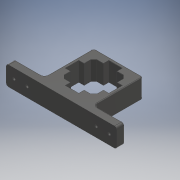
# Autodesk Inventor part: Support moteur
Saved by Autodesk Inventor 2017 (Build 210142000, 142)
## iProperties
Company: FABLAB Frenchmakers
Part Number: Support moteur
Material: Plastique ABS
Document SubType Name: Modeling
Designer: FABLAB Frenchmakers
Density: 1.06 g/cm^3
Appearance: Lisse - Blanc(3)
Mass: 88.0061 g
Surface Area: 230.451 cm^2
Volume: 83.0246 cm^3
Project: 1420 Vauban 3D XL
Catalog Web Link: http://frenchmakers.com/
Stock Number: 1420-05-01
Autodesk Inventor part; units mm, degrees
ref_plane "YZ Plane" through (0, 0, 0) normal (1, 0, 0) x (0, 1, 0)
ref_plane "XZ Plane" through (0, 0, 0) normal (0, 1, 0) x (-1, 0, 0)
sketch "Esquisse1" plane through (0, 0, 0) normal (0, 0, 1) x (1, 0, 0)
  line L0 (-17.3, -21.3) -> (17.3, -21.3)
  line L1 (21.3, -17.3) -> (21.3, 17.3)
  line L2 (17.3, 21.3) -> (-17.3, 21.3)
  line L3 (-21.3, 17.3) -> (-21.3, -17.3)
  line L4 (-21.3, -21.3) -> (21.3, 21.3) construction
  line L5 (21.3, -21.3) -> (-21.3, 21.3) construction
  line L6 (-21.3, 17.3) -> (-17.3, 21.3)
  line L7 (21.3, 17.3) -> (17.3, 21.3)
  line L8 (21.3, -17.3) -> (17.3, -21.3)
  line L9 (-17.3, -21.3) -> (-21.3, -17.3)
  line L10 (-32.3, -32.3) -> (32.3, -32.3)
  line L11 (32.3, -32.3) -> (32.3, 32.3)
  line L12 (32.3, 32.3) -> (-32.3, 32.3)
  line L13 (-32.3, 32.3) -> (-32.3, -32.3)
  line L14 (-32.3, -32.3) -> (32.3, 32.3) construction
  line L15 (32.3, -32.3) -> (-32.3, 32.3) construction
  point P0 (0, 0)
  dimension "d0" = 42.6
  dimension "d1" = 42.6
  dimension "d7" = 4
  dimension "d8" = 4
  dimension "d9" = 4
  dimension "d10" = 4
  dimension "d11" = 4
  dimension "d12" = 4
  dimension "d13" = 4
  dimension "d14" = 4
  dimension "d15" = 11
  dimension "d16" = 11
  constraints: 32 end point, 8 point on line, 4 midpoint, 4 parallel, 2 horizontal, 2 perpendicular
  measures "d0" distance of L5.end L4.end
  measures "d1" distance of L4.end L5.start
  measures "d7" distance of L3.start L5.end
  measures "d8" distance of L2.end L5.end
  measures "d9" distance of L1.end L4.end
  measures "d10" distance of L2.start L4.end
  measures "d11" distance of L1.start L5.start
  measures "d12" distance of L0.end L5.start
  measures "d13" distance of L0.start L4.start
  measures "d14" distance of L3.end L4.start
  measures "d15" distance between parallel lines of L2 L12
  measures "d16" distance between parallel lines of L3 L13
extrude "Extrusion1" add sketch "Esquisse1" along normal mid plane 25
sketch "Esquisse2" plane through (-32.3, -32.3, 12.5) normal (0, -1, 0) x (1, 0, 0)
  line L0 (-40, 0) -> (104.6, 0)
  line L1 (104.6, 0) -> (104.6, -25)
  line L2 (104.6, -25) -> (-40, -25)
  line L3 (-40, -25) -> (-40, 0)
  line L4 (-40, 0) -> (104.6, -25) construction
  line L5 (104.6, 0) -> (-40, -25) construction
  line L6 (0, 0) -> (64.6, 0) projected
  line L7 (64.6, -25) -> (64.6, 0) projected
  point P0 (32.3, -12.5)
  dimension "d17" = 40
  constraints: 12 end point, 2 midpoint, 2 parallel, 1 collinear, 1 horizontal, 1 perpendicular
  measures "d17" distance between parallel lines of L7 L1
extrude "Extrusion2" add sketch "Esquisse2" along normal blind 10
sketch "Esquisse3" plane through (-32.3, -32.3, 12.5) normal (0, 1, 0) x (1, 0, 0)
  line L0 (64.6, 0) -> (104.6, 0) construction
  line L1 (-40, 0) -> (0, 0) construction
  line L2 (-40, 25) -> (-40, 0) construction
  line L3 (104.6, 0) -> (104.6, 25) projected
  line L4 (64.6, 25) -> (64.6, 0) projected
  line L5 (0, 25) -> (0, 0) projected
  point P0 (32.3, 12.5)
  point P1 (77.6, 12.5)
  point P2 (-13, 12.5)
  point P3 (84.6, 0)
  point P4 (-20, 0)
  point P5 (-40, 12.5)
  point P6 (94.6, 12.5)
  point P7 (-30, 12.5)
  dimension "d31" = 20
  dimension "d32" = 20
  dimension "d33" = 7
  dimension "d34" = 10
  dimension "d35" = 20
  dimension "d36" = 20
  dimension "d37" = 10
  dimension "d38" = 7
  constraints: 4 horizontal alignment, 3 midpoint
  measures "d31" distance from line of L4 point (84.6, 0)
  measures "d32" distance from line of L3 point (84.6, 0)
  measures "d33" horizontal distance of point (84.6, 0) point (77.6, 12.5)
  measures "d34" horizontal distance of point (84.6, 0) point (94.6, 12.5)
  measures "d35" distance from line of point (-20, 0) L5
  measures "d36" distance from line of L2 point (-20, 0)
  measures "d37" horizontal distance of point (-20, 0) point (-30, 12.5)
  measures "d38" horizontal distance of point (-20, 0) point (-13, 12.5)
hole "Perçage1" at (45.3, -32.3, 0) at (-45.3, -32.3, 0) at (62.3, -32.3, 0) at (-62.3, -32.3, 0) direction (0, -1, 0) diameter 3.5 end through all counterbore diameter 6.5 counterbore depth 4
fillet "Congé1" radius 3 6 edges at (72.3, -37.3, -12.5) (72.3, -37.3, 12.5) (32.3, 32.3, 0) (-32.3, 32.3, 0) (-72.3, -37.3, -12.5) (-72.3, -37.3, 12.5)
fillet "Congé1" radius 5 2 edges at (-32.3, -32.3, 0) (32.3, -32.3, 0)
sketch "Esquisse4" plane through (0, 0, -12.5) normal (0, 0, -1) x (-1, 0, 0)
  line L0 (-17.3, -21.3) -> (17.3, -21.3) projected
  line L1 (8.625, -28.3) -> (-8.625, -28.3)
  line L2 (-8.625, -28.3) -> (-8.625, -21.3)
  line L3 (-8.625, -21.3) -> (8.625, -21.3)
  line L4 (8.625, -21.3) -> (8.625, -28.3)
  point P0 (0, 0)
  dimension "d39" = 17.25
  dimension "d40" = 8.625
  dimension "d41" = 7
  constraints: 8 end point, 2 parallel, 1 horizontal, 1 perpendicular, 1 point on line
  measures "d39" distance between parallel lines of L2 L4
  measures "d40" distance from line of point (0, 0) L2
  measures "d41" distance between parallel lines of L0 L1
extrude "Extrusion3" cut sketch "Esquisse4" against normal through all
ref_plane "Plan de construction1" through (0, -17.3, -12.5) normal (1, 0, 0) x (0, 0, -1)
pattern_circular "Réseau circulaire2" count 4 over 360 about axis through (0, 0, -10) along (0, 0, 1) of "Extrusion3"
fillet "Congé2" radius 1 24 edges at (-32.3, 1, 12.5) (-31.4213, 31.4213, 12.5) (0, 32.3, 12.5) (31.4213, 31.4213, 12.5) (32.3, 1, 12.5) (33.7645, -30.8355, 12.5) (-53.3, -32.3, 12.5) (53.3, -32.3, 12.5) (71.4213, -32.3, 11.6213) (72.3, -32.3, 0) (71.4213, -32.3, -11.6213) (-53.3, -32.3, -12.5) (53.3, -32.3, -12.5) (33.7645, -30.8355, -12.5) (32.3, 1, -12.5) (31.4213, 31.4213, -12.5) (0, 32.3, -12.5) (-31.4213, 31.4213, -12.5) (-32.3, 1, -12.5) (-33.7645, -30.8355, -12.5) (-71.4213, -32.3, -11.6213) (-72.3, -32.3, 0) (-71.4213, -32.3, 11.6213) (-33.7645, -30.8355, 12.5)
chamfer "Chanfrein2" distance 0.25 angle 45 60 edges at (-62.3, -42.3, -1.75) (-45.3, -42.3, -1.75) (45.3, -42.3, -1.75) (62.3, -42.3, -1.75) (45.3, -36.3, -1.75) (62.3, -36.3, -1.75) (-45.3, -36.3, -1.75) (-62.3, -36.3, -1.75) (-62.3, -32.3, -3.25) (-45.3, -32.3, -3.25) (62.3, -32.3, -3.25) (45.3, -32.3, -3.25) (-8.625, -24.8, 12.5) (-12.9625, -21.3, 12.5) (-19.3, -19.3, 12.5) (-21.3, -12.9625, 12.5) (-24.8, -8.625, 12.5) (-28.3, 0, 12.5) (-24.8, 8.625, 12.5) (-21.3, 12.9625, 12.5) (-8.625, 24.8, 12.5) (0, 28.3, 12.5) (8.625, 24.8, 12.5) (-12.9625, 21.3, 12.5) (-19.3, 19.3, 12.5) (0, -28.3, 12.5) (8.625, -24.8, 12.5) (12.9625, -21.3, 12.5) (19.3, -19.3, 12.5) (21.3, -12.9625, 12.5) (24.8, -8.625, 12.5) (28.3, 0, 12.5) (24.8, 8.625, 12.5) (21.3, 12.9625, 12.5) (19.3, 19.3, 12.5) (12.9625, 21.3, 12.5) (24.8, -8.625, -12.5) (21.3, -12.9625, -12.5) (19.3, -19.3, -12.5) (12.9625, -21.3, -12.5) (8.625, -24.8, -12.5) (0, -28.3, -12.5) (-8.625, -24.8, -12.5) (-12.9625, -21.3, -12.5) (-19.3, -19.3, -12.5) (-21.3, -12.9625, -12.5) (-24.8, -8.625, -12.5) (28.3, 0, -12.5) (24.8, 8.625, -12.5) (21.3, 12.9625, -12.5) (-28.3, 0, -12.5) (-24.8, 8.625, -12.5) (-21.3, 12.9625, -12.5) (-19.3, 19.3, -12.5) (-12.9625, 21.3, -12.5) (-8.625, 24.8, -12.5) (0, 28.3, -12.5) (8.625, 24.8, -12.5) (12.9625, 21.3, -12.5) (19.3, 19.3, -12.5)
equation "\"d1\" = d0"
equation "\"d8\" = d7"
equation "\"d9\" = d7"
equation "\"d10\" = d9"
equation "\"d11\" = d7"
equation "\"d12\" = d11"
equation "\"d13\" = d7"
equation "\"d14\" = d13"
equation "\"d16\" = d15"
equation "\"d34\" = 0.5 * d32"
equation "\"d37\" = d34"
equation "\"d38\" = d33"
equation "\"d40\" = 0.5 * d39"
